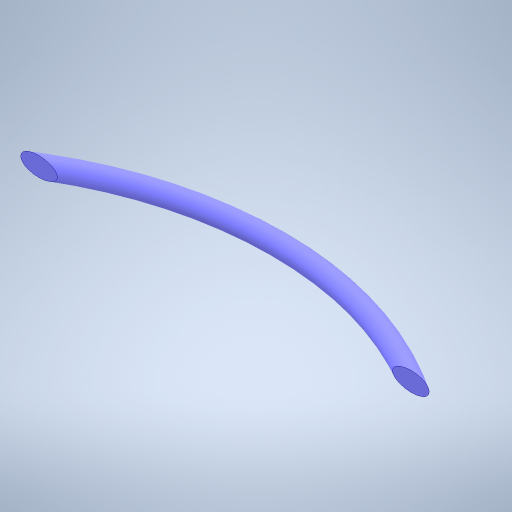
# Autodesk Inventor part: Hula Hoop-1
Saved by Autodesk Inventor 2024 (Build 280153000, 153)
## iProperties
Created: 2024-03-21
Part Number: Hula Hoop-1
Material: Generic
Document SubType Name: Modeling
Designer: anyangoe
Density: 1 g/cm^3
Appearance: Default
Author: anyangoe
Autodesk Inventor part; units mm, degrees
ref_plane "YZ Plane" through (0, 0, 0) normal (1, 0, 0) x (0, 1, 0)
ref_plane "XZ Plane" through (0, 0, 0) normal (0, 1, 0) x (-1, 0, 0)
ref_plane "XY Plane" through (0, 0, 0) normal (0, 0, 1) x (1, 0, 0)
sketch "Sketch1" plane through (0, 0, 0) normal (1, 0, 0) x (0, 1, 0)
  circle A0 centre (0, -355.6) radius 9.525
  line L0 (-13.335, 0) -> (13.335, 0) projected
  point P0 (0, 0)
  dimension "d0" = 19.05
  dimension "d1" = 355.6
  constraints: 1 centre point, 1 vertical alignment
  measures "d0" diameter of A0
  measures "d1" distance of point (0, 0) A0.centre
revolve "Revolution1" add sketch "Sketch1" angle 360 about axis through (0, -10, 0) along (0, 1, 0)
sketch "Sketch2" plane through (0, 0, 0) normal (0, 1, 0) x (-1, 0, 0)
  circle A0 centre (0, 0) radius 365.125 projected
  line L0 (203.2, -303.3579) -> (-203.2, -303.3579)
  dimension "d3" = 406.4
  constraints: 2 end point, 2 point on circle, 1 horizontal
  measures "d3" distance of L0.start L0.end
extrude "Extrusion1" cut sketch "Sketch2" along normal mid plane 25.4 contours A0 L0 picked at (3.0391, -80.5682)
body "Solid1"
